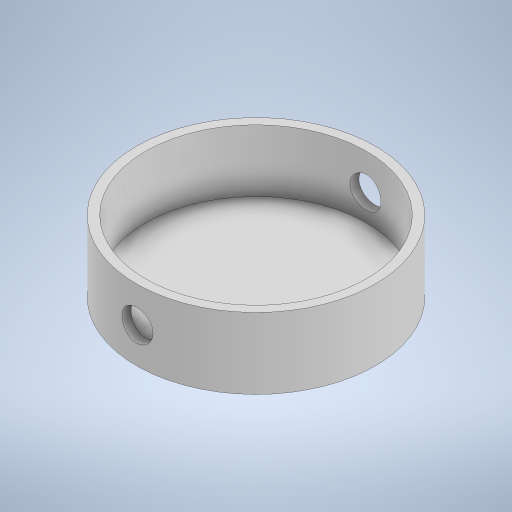
# Autodesk Inventor part: UpstreamVolume
Saved by Autodesk Inventor 2023 (Build 270158000, 158)
## iProperties
Created: 2023-01-27
Part Number: UpstreamVolume
Material: Generic
Document SubType Name: Modeling
Designer: remidm
Density: 1 g/cm^3
Appearance: Default
Author: remidm
Autodesk Inventor part; units mm, degrees
ref_plane "YZ Plane" through (0, 0, 0) normal (1, 0, 0) x (0, 1, 0)
ref_plane "XZ Plane" through (0, 0, 0) normal (0, 1, 0) x (-1, 0, 0)
ref_plane "XY Plane" through (0, 0, 0) normal (0, 0, 1) x (1, 0, 0)
sketch "Sketch1" plane through (0, 0, 0) normal (0, 0, 1) x (1, 0, 0)
  line L0 (-25, 0) -> (-25, 14.0559)
  line L1 (-27, 14.0559) -> (-27, -2)
  line L2 (-25, 0) -> (0, 0)
  line L3 (0, 0) -> (0, -2)
  line L4 (0, -2) -> (-27, -2)
  line L5 (0, -422005.1648) -> (0, 70350.5927) projected
  arc A0 (-25, 14.0559) -> (-27, 14.0559) centre (-27, -351668.6281) ccw
  dimension "d5" = 2
  dimension "radius" = 25
  dimension "d7" = 2
  constraints: 10 end point, 2 perpendicular, 2 point on circle, 1 centre point, 1 horizontal, 1 point on line, 1 vertical
  measures "d5" distance between parallel lines of L4 L2
  measures "radius" distance from line of L2.end L0
  measures "d7" distance between parallel lines of L0 L1
revolve "Revolution1" add sketch "Sketch1" angle 360 about axis through (0, -10, 0) along (0, 1, 0)
sketch "Sketch4" plane through (0, 0, 0) normal (0, 0, 1) x (1, 0, 0)
  line L0 (40.24, 12) -> (-40.24, 12) projected
  line L1 (0, 0) -> (0, 6)
  line L2 (0, 6) -> (0, 12)
  constraints: 4 end point, 1 collinear, 1 midpoint, 1 vertical
hole "Hole3" at (0, 6, 0) direction (0, 0, -1) diameter 7 end through all both
equation "\"d30\" = PenetrationUpstreamInnerDiameter + 2 * PenetrationUpstreamThickness"
equation "\"d5\" = thickness"
equation "\"radius\" = 0.5 * SaltDiameter"
equation "\"d7\" = thickness"
equation "\"thickness\" = crucible_thickness"
equation "\"CrucibleHeightBelowMembrane\" = 14"
equation "\"PenetrationUpstreamInnerDiameter\" = 5"
equation "\"PenetrationUpstreamThickness\" = 1"
equation "\"SaltDiameter\" = 50"
equation "\"crucible_thickness\" = 2"
body "Solid1"
